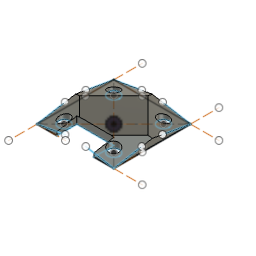
ecen240_mount (Autodesk Fusion 360 design; units mm, degrees)
Autodesk Fusion 360 part; units mm, degrees
sketch "Sketch1" plane through (0, 0, 0) normal (0, 0, 1) x (1, 0, 0)
  line L0 (-13.5, -13.5) -> (-13.5, 13.5)
  line L1 (-13.5, 13.5) -> (13.5, 13.5)
  line L2 (13.5, 13.5) -> (13.5, -13.5)
  line L3 (13.5, -13.5) -> (-13.5, 13.5) construction
  line L4 (8.75, -8.75) -> (-8.75, 8.75) construction
  line L5 (-8.75, -8.75) -> (8.75, 8.75) construction
  circle A0 centre (-8.75, 8.75) radius 2
  circle A1 centre (8.75, 8.75) radius 2
  circle A2 centre (-8.75, -8.75) radius 2
  circle A3 centre (8.75, -8.75) radius 2
  line L6 (-13.5, -13.5) -> (7.3358, 7.3358) construction
  line L7 (8.75, 8.75) -> (13.5, 13.5) construction
  line L8 (-6.5, -13.5) -> (-6.5, -6.5)
  line L9 (-6.5, -6.5) -> (6.5, -6.5)
  line L10 (6.5, -6.5) -> (6.5, -13.5)
  line L11 (13.5, -13.5) -> (6.5, -13.5)
  line L12 (-6.5, -13.5) -> (-13.5, -13.5)
  dimension "d1" = 27
  dimension "d2" = 27
  dimension "d3" = 17.5
  dimension "d4" = 17.5
  dimension "d5" = 4
  dimension "d6" = 4
  dimension "d7" = 4
  dimension "d8" = 4
  dimension "d9" = 13
  constraint horizontal L11
  constraint perpendicular L0 L11
  constraint parallel L1 L11
  constraint parallel L0 L2
  constraint coincident L3 origin
  constraint coincident origin L6
  constraint coincident L4 origin
  constraint coincident L5 origin
  constraint coincident L4.end A0.centre
  constraint coincident L5.end A1.centre
  constraint coincident L5.start A2.centre
  constraint coincident L4.start A3.centre
  constraint coincident A1 L6.end
  constraint collinear L6 L7
  constraint parallel L8 L10
  constraint coincident L8.start L11
  constraint collinear L11 L12
  measures "d1" distance of L0.end L1.end
  measures "d2" distance of L0.start L0.end
  measures "d3" distance of L4.end L5.end
  measures "d4" distance of L5.start L4.end
  measures "d5" diameter of A0
  measures "d6" diameter of A1
  measures "d7" diameter of A2
  measures "d8" diameter of A3
  measures "d9" distance of L8.end L9.end
ref_plane "WorkPlane1" through (13.5, 0, 0) normal (1, 0, 0) x (0, 1, 0)
ref_plane "WorkPlane2" through (-13.5, 0, 0) normal (1, 0, 0) x (0, 1, 0)
ref_plane "WorkPlane3" through (13.5, 0, 0) normal (1, 0, 0) x (0, 1, 0)
sketch "Sketch4" plane through (13.5, 0, 0) normal (1, 0, 0) x (0, 1, 0)
  line L0 (-13.5, 0) -> (-3.6519, 1.7365)
  line L1 (-13.5, 0) -> (-3.5, 0) construction
  line L2 (13.5, 0) -> (3.6519, 1.7365)
  line L3 (13.5, 0) -> (23.5, 0) construction
  dimension "d22" = 10
  dimension "d23" = 10
  dimension "d24" = 170
  dimension "d25" = 10
  constraint horizontal L1
  constraint horizontal L3
  measures "d22" distance of L0.start L0.end
  measures "d23" angle of L0 L1
  measures "d24" angle of L2 L3
  measures "d25" distance of L2.start L2.end
ref_plane "WorkPlane4" through (0, 13.5, 0) normal (0, 1, 0) x (0, 0, 1)
sketch "Sketch5" plane through (0, 13.5, 0) normal (0, 1, 0) x (1, 0, 0)
  line L0 (-13.5, 0) -> (-3.6519, -1.7365)
  line L1 (-13.5, 0) -> (-3.5, 0) construction
  line L2 (13.5, 0) -> (3.6519, -1.7365)
  line L3 (13.5, 0) -> (23.5, 0) construction
  dimension "d27" = 10
  dimension "d28" = 10
  dimension "d29" = 170
  dimension "d30" = 10
  constraint horizontal L1
  constraint horizontal L3
  measures "d27" angle of L0 L1
  measures "d28" distance of L0.start L0.end
  measures "d29" angle of L2 L3
  measures "d30" distance of L2.start L2.end
ref_plane "WorkPlane5" through (0, -13.5, 0) normal (0, 1, 0) x (0, 0, 1)
sketch "Sketch6" plane through (0, -13.5, 0) normal (0, 1, 0) x (1, 0, 0)
  line L0 (-13.5, 0) -> (-3.6519, -1.7365)
  line L1 (-13.5, 0) -> (-3.5, 0) construction
  line L2 (13.5, 0) -> (3.6519, -1.7365)
  line L3 (13.5, 0) -> (23.5, 0) construction
  dimension "d32" = 10
  dimension "d33" = 10
  dimension "d34" = 170
  dimension "d35" = 10
  constraint horizontal L1
  constraint horizontal L3
  measures "d32" distance of L0.start L0.end
  measures "d33" angle of L0 L1
  measures "d34" angle of L2 L3
  measures "d35" distance of L2.start L2.end
extrude "Extrude1" add sketch "Sketch1" along normal blind 2.64 makes body 1
ref_plane "WorkPlane6" through (13.5, -13.5, 0) normal (-0.171088, 0.171088, -0.970288) x (-0.707107, -0.707107, 0)
ref_plane "WorkPlane7" through (13.5, 13.5, 0) normal (-0.171088, -0.171088, -0.970288) x (0.707107, -0.707107, 0)
ref_plane "WorkPlane8" through (0, 0, 0) normal (1, 0, 0) x (0, 1, 0)
ref_plane "WorkPlane9" through (-13.5, 0, 0) normal (1, 0, 0) x (0, 1, 0)
sketch "Sketch7" plane through (-13.5, 0, 0) normal (1, 0, 0) x (0, 1, 0)
  line L0 (13.5, 0) -> (23.5, 0) construction
  line L1 (13.5, 0) -> (3.6519, 1.7365)
  line L2 (13.5, 0) -> (3.5, 0) construction
  line L3 (-13.5, 0) -> (-3.6519, 1.7365)
  line L4 (-13.5, 0) -> (-23.5, 0) construction
  dimension "d43" = 10
  dimension "d44" = 10
  dimension "d45" = 10
  dimension "d46" = 170
  constraint horizontal L0
  constraint horizontal L2
  constraint horizontal L4
  measures "d43" angle of L1 L2
  measures "d44" distance of L0.start L1.end
  measures "d45" distance of L3.start L3.end
  measures "d46" angle of L3 L4
ref_plane "WorkPlane10" through (-13.5, -13.5, 0) normal (-0.171088, -0.171088, 0.970288) x (0.707107, -0.707107, 0)
ref_plane "WorkPlane11" through (-13.5, 13.5, 0) normal (-0.171088, 0.171088, 0.970288) x (-0.707107, -0.707107, 0)
split "Split1" by plane through (13.5, 13.5, 0) normal (-0.171088, -0.171088, -0.970288) bodies 1 makes body 2 at (-2.1667, 2.7598, 0)
delete_body "RemoveBody1" bodies 1
split "Split2" by plane through (-13.5, -13.5, 0) normal (-0.171088, -0.171088, 0.970288) bodies 2 makes body 3 at (-12.5759, -6.8266, 2.64)
delete_body "RemoveBody2" bodies 3
split "Split3" by plane through (13.5, -13.5, 0) normal (-0.171088, 0.171088, -0.970288) bodies 2 makes body 4 at (-2.1667, 2.7598, 0)
delete_body "RemoveBody3" bodies 2
split "Split4" by plane through (-13.5, 13.5, 0) normal (-0.171088, 0.171088, 0.970288) bodies 4 makes body 5 at (-12.5759, 7.808, 2.64)
delete_body "RemoveBody4" bodies 5
